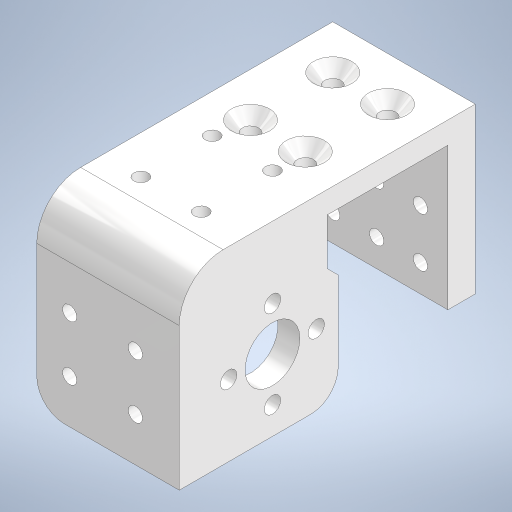
# Autodesk Inventor part: probe_block_R
Saved by Autodesk Inventor 2024.1 (Build 281209000, 209)
## iProperties
Created: 2023-08-28
Part Number: probe_block_R
Material: ABS Plastic
Document SubType Name: Modeling
Designer: l1534
Density: 1.06 g/cm^3
Appearance: Smooth - White
Author: l1534
Autodesk Inventor part; units mm, degrees
ref_plane "YZ Plane" through (0, 0, 0) normal (1, 0, 0) x (0, 1, 0)
ref_plane "XZ Plane" through (0, 0, 0) normal (0, 1, 0) x (-1, 0, 0)
ref_plane "XY Plane" through (0, 0, 0) normal (0, 0, 1) x (1, 0, 0)
sketch "Sketch1" plane through (0, 0, 0) normal (0, 1, 0) x (-1, 0, 0)
  line L0 (-12.6881, -33.1691) -> (13.3119, -33.1691)
  line L1 (13.3119, -33.1691) -> (13.3119, 11.8309)
  line L2 (13.3119, 11.8309) -> (-12.6881, 11.8309)
  line L3 (-12.6881, 11.8309) -> (-12.6881, -33.1691)
  point P0 (0, 0)
  dimension "d0" = 45
  dimension "d1" = 26
  constraints: 8 end point, 2 parallel, 1 horizontal, 1 perpendicular
  measures "d0" distance of L2.end L0.start
  measures "d1" distance of L1.end L2.end
extrude "Extrusion1" add sketch "Sketch1" along normal blind 4
sketch "Sketch2" plane through (0, 0, 0) normal (0, -1, 0) x (1, 0, 0)
  line L0 (-13.3119, 11.8309) -> (12.6881, 11.8309) projected
  line L1 (12.6881, 11.8309) -> (8.6881, 11.8309)
  line L2 (8.6881, 11.8309) -> (8.6881, -13.1691)
  line L3 (8.6881, -13.1691) -> (12.6881, -13.1691)
  line L4 (12.6881, -13.1691) -> (12.6881, 11.8309)
  point P0 (0, 0)
  point P1 (10.6881, -13.1691)
  dimension "d4" = 4
  dimension "d5" = 25
  constraints: 8 end point, 2 parallel, 1 horizontal, 1 midpoint, 1 perpendicular
  measures "d4" distance between parallel lines of L4 L2
  measures "d5" distance from line of L0 point (10.688, -13.169)
extrude "Extrusion2" add sketch "Sketch2" along normal blind 30
sketch "Sketch4" plane through (8.6881, 0, -13.1691) normal (-1, 0, 0) x (0, 0, 1)
  circle A0 centre (12, -17) radius 5
  line L0 (25, -30) -> (0, -30) projected
  line L1 (25, 0) -> (25, -30) projected
  point P0 (13.1691, 0)
  dimension "d8" = 10
  dimension "d9" = 13
  dimension "d10" = 13
  constraints: 1 centre point
  measures "d8" diameter of A0
  measures "d9" distance from line of L0 A0.centre
  measures "d10" distance from line of L1 A0.centre
extrude "Extrusion3" cut sketch "Sketch4" against normal through all
sketch "Sketch5" plane through (8.6881, 0, -13.1691) normal (-1, 0, 0) x (0, 0, 1)
  circle A0 centre (12, -9) radius 1.5
  circle A1 centre (12, -25) radius 1.5
  circle A2 centre (20, -17) radius 1.5
  circle A3 centre (4, -17) radius 1.5
  circle A4 centre (12, -17) radius 5 projected
  point P0 (13.1691, 0)
  dimension "d13" = 3
  dimension "d14" = 3
  dimension "d15" = 3
  dimension "d16" = 3
  dimension "d17" = 8
  dimension "d19" = 8
  dimension "d20" = 8
  dimension "d21" = 8
  dimension "d22" = 8
  dimension "d23" = 8
  dimension "d24" = 8
  constraints: 4 centre point
  measures "d13" diameter of A0
  measures "d14" diameter of A2
  measures "d15" diameter of A3
  measures "d16" diameter of A1
  measures "d17" distance of A4.centre A1.centre
  measures "d19" distance of A4.centre A3.centre
  measures "d20" distance of A4.centre A0.centre
  measures "d21" distance of A4.centre A2.centre
  measures "d22" horizontal distance of A1.centre A2.centre
  measures "d23" horizontal distance of A1.centre A3.centre
  measures "d24" horizontal distance of A2.centre A0.centre
extrude "Extrusion4" cut sketch "Sketch5" against normal through all contours A0 | A1 | A2 | A3
sketch "Sketch9" plane through (-13.3119, 4, 11.8309) normal (0, 0, 1) x (1, 0, 0)
  line L0 (0, -4) -> (0, 0) projected
  line L1 (26, -4) -> (26, -34) projected
  line L2 (0, 0) -> (26, 0)
  line L3 (26, 0) -> (26, -34)
  line L4 (26, -34) -> (0, -34)
  line L5 (0, -34) -> (0, 0)
  point P0 (13.3119, -4)
  constraints: 8 end point, 2 parallel, 1 horizontal, 1 perpendicular
extrude "Extrusion6" add sketch "Sketch9" along normal blind 4
fillet "Fillet3" radius 5 3 edges at (-13.3119, -30, 13.8309) (10.6881, -30, -13.1691) (-2.3119, 0, 11.8309)
fillet "Fillet4" radius 8 1 edges at (-0.3119, 4, 15.8309)
fillet "Fillet5" radius 1.5 3 edges at (8.6881, -1.4645, 10.3664) (8.6881, 0, -3.1691) (8.6881, -17.5, 11.8309)
sketch "Sketch10" plane through (12.6881, 0, -33.1691) normal (0, 0, -1) x (-1, 0, 0)
  line L0 (0, 4) -> (26, 4) projected
  line L1 (0, 4) -> (26, 4)
  line L2 (26, 4) -> (26, -26)
  line L3 (26, -26) -> (0, -26)
  line L4 (0, -26) -> (0, 4)
  point P0 (12.6881, 0)
  dimension "d44" = 30
  constraints: 8 end point, 2 parallel, 1 horizontal, 1 perpendicular
  measures "d44" distance of L1.end L2.end
extrude "Extrusion7" add sketch "Sketch10" along normal blind 5
sketch "Sketch12" plane through (12.6881, 0, -38.1691) normal (0, 0, -1) x (-1, 0, 0)
  circle A0 centre (5, -3) radius 1.3
  circle A1 centre (21, -3) radius 1.3
  circle A2 centre (5, -21) radius 1.3
  circle A3 centre (21, -21) radius 1.3
  circle A4 centre (21, -12) radius 1.3
  line L0 (26, -26) -> (26, 4) projected
  line L1 (0, 4) -> (0, -26) projected
  line L2 (26, 4) -> (0, 4) projected
  line L3 (0, -26) -> (26, -26) projected
  circle A5 centre (5, -12) radius 1.3
  circle A6 centre (13, -21) radius 1.3
  circle A7 centre (13, -12) radius 1.3
  circle A8 centre (13, -3) radius 1.3
  point P0 (12.6881, 0)
  dimension "d47" = 2.6
  dimension "d48" = 2.6
  dimension "d49" = 2.6
  dimension "d50" = 2.6
  dimension "d51" = 2.6
  dimension "d52" = 5
  dimension "d53" = 5
  dimension "d54" = 5
  dimension "d55" = 5
  dimension "d56" = 7
  dimension "d57" = 7
  dimension "d58" = 16
  dimension "d59" = 5
  dimension "d60" = 5
  dimension "d61" = 5
  dimension "d64" = 2.6
  dimension "d65" = 16
  dimension "d66" = 5
  dimension "d81" = 2.6
  dimension "d82" = 2.6
  dimension "d83" = 2.6
  dimension "d84" = 5
  dimension "d85" = 13
  dimension "d86" = 13
  dimension "d87" = 13
  dimension "d88" = 7
  dimension "d89" = 16
  constraints: 9 centre point
  measures "d47" diameter of A4
  measures "d48" diameter of A0
  measures "d49" diameter of A1
  measures "d50" diameter of A2
  measures "d51" diameter of A3
  measures "d52" distance from line of L0 A1.centre
  measures "d53" distance from line of L1 A0.centre
  measures "d54" distance from line of L1 A2.centre
  measures "d55" distance from line of L0 A3.centre
  measures "d56" distance from line of L2 A1.centre
  measures "d57" distance from line of L2 A0.centre
  measures "d58" distance from line of L2 A4.centre
  measures "d59" distance from line of L0 A4.centre
  measures "d60" distance from line of L3 A2.centre
  measures "d61" distance from line of L3 A3.centre
  measures "d64" diameter of A5
  measures "d65" distance from line of L2 A5.centre
  measures "d66" distance from line of L1 A5.centre
  measures "d81" diameter of A8
  measures "d82" diameter of A7
  measures "d83" diameter of A6
  measures "d84" distance from line of L3 A6.centre
  measures "d85" distance from line of L0 A6.centre
  measures "d86" distance from line of L0 A7.centre
  measures "d87" distance from line of L0 A8.centre
  measures "d88" distance from line of L2 A8.centre
  measures "d89" distance from line of L2 A7.centre
extrude "Extrusion8" cut sketch "Sketch12" against normal up to surface (5 mm away) contours A0 | A1 | A2 | A3 | A4 | A5 | A6 | A7 | A8
sketch "Sketch13" plane through (0, 4, 0) normal (0, 1, 0) x (1, 0, 0)
  circle A0 centre (4.6881, 30.1691) radius 1.5
  circle A1 centre (4.6881, 15.1691) radius 1.5
  circle A2 centre (-5.3119, 30.1691) radius 1.5
  circle A3 centre (-5.3119, 15.1691) radius 1.5
  line L0 (-13.3119, 38.1691) -> (12.6881, 38.1691) projected
  line L1 (12.6881, 38.1691) -> (12.6881, -7.8309) projected
  point P0 (0, 0)
  dimension "d67" = 3
  dimension "d68" = 3
  dimension "d69" = 3
  dimension "d70" = 3
  dimension "d71" = 10
  dimension "d72" = 15
  dimension "d73" = 15
  dimension "d74" = 8
  dimension "d75" = 8
  dimension "d76" = 8
  dimension "d77" = 8
  dimension "d78" = 10
  constraints: 4 centre point
  measures "d67" diameter of A0
  measures "d68" diameter of A1
  measures "d69" diameter of A2
  measures "d70" diameter of A3
  measures "d71" distance of A2.centre A0.centre
  measures "d72" distance of A1.centre A0.centre
  measures "d73" distance of A2.centre A3.centre
  measures "d74" distance from line of L0 A0.centre
  measures "d75" distance from line of L0 A2.centre
  measures "d76" distance from line of L1 A0.centre
  measures "d77" distance from line of L1 A1.centre
  measures "d78" distance of A1.centre A3.centre
extrude "Extrusion9" cut sketch "Sketch13" against normal through all
chamfer "Chamfer3" distance 2 angle 45 4 edges at (3.1881, 4, -30.1691) (-6.8119, 4, -30.1691) (3.1881, 4, -15.1691) (-6.8119, 4, -15.1691)
sketch "Sketch14" plane through (-13.3119, 4, 15.8309) normal (0, 0, 1) x (1, 0, 0)
  circle A0 centre (6, -16) radius 1.3
  circle A1 centre (18, -16) radius 1.3
  circle A2 centre (6, -26) radius 1.3
  circle A3 centre (18, -26) radius 1.3
  line L0 (26, -34) -> (26, -8) projected
  line L1 (0, -8) -> (0, -29) projected
  line L2 (5, -34) -> (26, -34) projected
  point P0 (13.3119, -4)
  dimension "d93" = 2.6
  dimension "d94" = 2.6
  dimension "d95" = 2.6
  dimension "d96" = 2.6
  dimension "d97" = 8
  dimension "d98" = 8
  dimension "d99" = 6
  dimension "d100" = 6
  dimension "d101" = 8
  dimension "d102" = 8
  dimension "d103" = 10
  dimension "d104" = 10
  constraints: 4 centre point
  measures "d93" diameter of A0
  measures "d94" diameter of A1
  measures "d95" diameter of A2
  measures "d96" diameter of A3
  measures "d97" distance from line of L0 A1.centre
  measures "d98" distance from line of L0 A3.centre
  measures "d99" distance from line of L1 A0.centre
  measures "d100" distance from line of L1 A2.centre
  measures "d101" distance from line of L2 A3.centre
  measures "d102" distance from line of L2 A2.centre
  measures "d103" distance of A2.centre A0.centre
  measures "d104" distance of A3.centre A1.centre
extrude "Extrusion10" cut sketch "Sketch14" against normal up to surface (4 mm away)
sketch "Sketch15" plane through (0, 4, 0) normal (0, 1, 0) x (1, 0, 0)
  circle A0 centre (-6.3119, 9.1691) radius 1.3
  circle A1 centre (-6.3119, -3.8309) radius 1.3
  circle A2 centre (4.6881, -3.8309) radius 1.3
  circle A3 centre (4.6881, 9.1691) radius 1.3
  line L0 (12.6881, 38.1691) -> (12.6881, -7.8309) projected
  line L1 (-13.3119, -7.8309) -> (-13.3119, 38.1691) projected
  line L2 (-13.3119, 38.1691) -> (12.6881, 38.1691) projected
  point P0 (0, 0)
  dimension "d107" = 2.6
  dimension "d108" = 2.6
  dimension "d109" = 2.6
  dimension "d110" = 2.6
  dimension "d111" = 8
  dimension "d112" = 8
  dimension "d113" = 7
  dimension "d114" = 7
  dimension "d115" = 13
  dimension "d116" = 13
  dimension "d117" = 29
  dimension "d118" = 29
  constraints: 4 centre point
  measures "d107" diameter of A3
  measures "d108" diameter of A2
  measures "d109" diameter of A0
  measures "d110" diameter of A1
  measures "d111" distance from line of L0 A3.centre
  measures "d112" distance from line of L0 A2.centre
  measures "d113" distance from line of L1 A0.centre
  measures "d114" distance from line of L1 A1.centre
  measures "d115" distance of A2.centre A3.centre
  measures "d116" distance of A1.centre A0.centre
  measures "d117" distance from line of L2 A3.centre
  measures "d118" distance from line of L2 A0.centre
extrude "Extrusion11" cut sketch "Sketch15" against normal up to surface (4 mm away)
sketch "Sketch18" plane through (12.6881, -25, -13.1691) normal (1, 0, 0) x (0, 0, -1)
  line L0 (-20, 25) -> (0, 25) projected
  line L1 (0, 25) -> (-2, 25)
  line L2 (-2, 25) -> (-2, 16.5)
  line L3 (-2, 16.5) -> (0, 16.5)
  line L4 (0, 16.5) -> (0, 25)
  point P0 (-13.1691, 25)
  point P1 (-2, 25)
  dimension "d124" = 8.5
  dimension "d125" = 2
  constraints: 8 end point, 2 parallel, 1 horizontal, 1 perpendicular
  measures "d124" distance of L3.end L0.end
  measures "d125" distance between parallel lines of L4 L2
extrude "Extrusion13" cut sketch "Sketch18" against normal through all
chamfer "Chamfer4" distance 2 angle 45 1 edges at (10.6881, -8.5, -13.1691)
equation "\"d78\" = d71"
body "Solid1"
